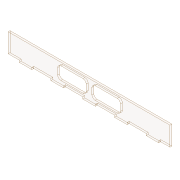
# Autodesk Inventor part: Divisória-25cm Frontal
Saved by Autodesk Inventor 2020 (Build 240168000, 168)
## iProperties
Created: 2021-09-22
Part Number: Divisória-25cm Frontal
Material: Generic
Document SubType Name: Modeling
Designer: pablo
Density: 1 g/cm^3
Appearance: Polycarbonate - Smoked
Mass: 31.9646 g
Surface Area: 171 cm^2
Volume: 31.9646 cm^3
Author: pablo
Autodesk Inventor part; units mm, degrees
ref_plane "YZ Plane" through (0, 0, 0) normal (1, 0, 0) x (0, 1, 0)
ref_plane "XZ Plane" through (0, 0, 0) normal (0, 1, 0) x (-1, 0, 0)
ref_plane "XY Plane" through (0, 0, 0) normal (0, 0, 1) x (1, 0, 0)
sketch "Sketch1" plane through (0, 0, 0) normal (0, 0, 1) x (1, 0, 0)
  line L0 (-127.5, 15) -> (127.5, 15)
  line L1 (127.5, 15) -> (127.5, -15)
  line L2 (127.5, -15) -> (-127.5, -15)
  line L3 (-127.5, -15) -> (-127.5, 15)
  line L4 (-127.5, 15) -> (127.5, -15) construction
  line L5 (127.5, 15) -> (-127.5, -15) construction
  point P0 (0, 0)
  dimension "d0" = 255
  dimension "d1" = 30
  constraints: 12 end point, 2 midpoint, 2 parallel, 1 horizontal, 1 perpendicular
  measures "d0" distance of L1.end L2.end
  measures "d1" distance of L0.end L1.end
extrude "Extrusion1" add sketch "Sketch1" along normal blind 3
sketch "Sketch2" plane through (0, 0, 3) normal (0, 0, 1) x (1, 0, 0)
  line L0 (-127.5, -15) -> (127.5, -15) projected
  line L1 (-110, -15) -> (-90, -15)
  line L2 (-90, -15) -> (-90, -18)
  line L3 (-90, -18) -> (-110, -18)
  line L4 (-110, -18) -> (-110, -15)
  line L5 (-60, -15) -> (-40, -15)
  line L6 (-40, -15) -> (-40, -18)
  line L7 (-40, -18) -> (-60, -18)
  line L8 (-60, -18) -> (-60, -15)
  line L9 (-10, -15) -> (10, -15)
  line L10 (10, -15) -> (10, -18)
  line L11 (10, -18) -> (-10, -18)
  line L12 (-10, -18) -> (-10, -15)
  line L13 (40, -15) -> (60, -15)
  line L14 (60, -15) -> (60, -18)
  line L15 (60, -18) -> (40, -18)
  line L16 (40, -18) -> (40, -15)
  line L17 (90, -15) -> (110, -15)
  line L18 (110, -15) -> (110, -18)
  line L19 (110, -18) -> (90, -18)
  line L20 (90, -18) -> (90, -15)
  point P0 (0, 0)
  point P1 (60, -15)
  point P2 (40, -15)
  point P3 (-90, -15)
  point P4 (-40, -15)
  point P5 (-60, -15)
  point P6 (10, -15)
  point P7 (-10, -15)
  point P8 (110, -15)
  point P9 (90, -15)
  dimension "d4" = 20
  dimension "d5" = 3
  dimension "d6" = 17.5
  dimension "d9" = 50
  dimension "d14" = 17.5
  constraints: 40 end point, 2 horizontal, 2 parallel, 1 collinear, 1 perpendicular, 1 point on line, 31 other
  measures "d4" distance of L2.end L3.end
  measures "d5" distance of L1.end L2.end
  measures "d6" horizontal distance of L3.end L0.start
  measures "d9" distance of L1.start L5.start
  measures "d14" horizontal distance of L18.end L0.end
extrude "Extrusion2" add sketch "Sketch2" against normal blind 3
sketch "Sketch3" plane through (0, 0, 3) normal (0, 0, 1) x (1, 0, 0)
  line L0 (9.5, 10) -> (44.5, 10)
  line L1 (49.5, 5) -> (49.5, -5)
  line L2 (44.5, -10) -> (9.5, -10)
  line L3 (4.5, -5) -> (4.5, 5)
  line L4 (4.5, 10) -> (49.5, -10) construction
  line L5 (49.5, 10) -> (4.5, -10) construction
  line L6 (0, -10) -> (0, 0)
  line L7 (-9.5, 10) -> (-44.5, 10)
  line L8 (-49.5, 5) -> (-49.5, -5)
  line L9 (-44.5, -10) -> (-9.5, -10)
  line L10 (-4.5, -5) -> (-4.5, 5)
  line L11 (-4.5, 10) -> (-49.5, -10) construction
  line L12 (-49.5, 10) -> (-4.5, -10) construction
  arc A0 (49.5, 5) -> (44.5, 10) centre (44.5, 5) ccw
  arc A1 (44.5, -10) -> (49.5, -5) centre (44.5, -5) ccw
  arc A2 (4.5, -5) -> (9.5, -10) centre (9.5, -5) ccw
  arc A3 (9.5, 10) -> (4.5, 5) centre (9.5, 5) ccw
  arc A4 (-4.5, 5) -> (-9.5, 10) centre (-9.5, 5) ccw
  arc A5 (-9.5, -10) -> (-4.5, -5) centre (-9.5, -5) ccw
  arc A6 (-44.5, 10) -> (-49.5, 5) centre (-44.5, 5) ccw
  arc A7 (-49.5, -5) -> (-44.5, -10) centre (-44.5, -5) ccw
  point P0 (27, 0)
  point P1 (-27, 0)
  dimension "d17" = 45
  dimension "d18" = 20
  dimension "d19" = 27
  dimension "d22" = 5
  constraints: 26 end point, 16 point on circle, 16 point on line, 16 tangent, 8 centre point, 7 equal radius, 5 symmetric about line, 4 midpoint, 2 parallel, 1 horizontal, 1 perpendicular, 1 vertical
  measures "d17" distance of L4.end L5.end
  measures "d18" distance of L5.start L4.end
  measures "d19" distance of L6.end point (27, 0)
  measures "d22" radius of A0
extrude "Extrusion3" cut sketch "Sketch3" against normal blind 3
body "Solid1"
